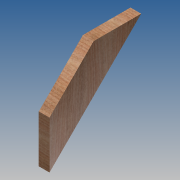
# Autodesk Inventor part: gableSupport
Saved by Autodesk Inventor 2013 (Build 170138000, 138)
## iProperties
Created: 2013-08-11
Part Number: gableSupport
Material: Wood (Birch)
Document SubType Name: Modeling
Designer: ddeboer
Mass: 2602.47 g
Surface Area: 2982.08 cm^2
Volume: 4731.76 cm^3
Density: 0.55 g/cm^3
Author: ddeboer
Autodesk Inventor part; units mm, degrees
ref_plane "YZ Plane" through (0, 0, 0) normal (1, 0, 0) x (0, 1, 0)
ref_plane "XZ Plane" through (0, 0, 0) normal (0, 1, 0) x (-1, 0, 0)
ref_plane "XY Plane" through (0, 0, 0) normal (0, 0, 1) x (1, 0, 0)
sketch "Sketch1" plane through (0, 0, 0) normal (1, 0, 0) x (0, 1, 0)
  line L0 (0, 0) -> (215.5261, -215.5261)
  line L1 (0, 0) -> (304.8, 0) construction
  line L2 (381, -183.4344) -> (337.2656, -139.7)
  line L3 (337.2656, -139.7) -> (197.5656, 0)
  line L4 (197.5656, 0) -> (0, 0)
  line L5 (215.5261, -215.5261) -> (381, -381)
  line L6 (381, -183.4344) -> (381, -381)
  dimension "d0" = 304.8
  dimension "d1" = 45
  dimension "d2" = 139.7
  dimension "d5" = 381
  constraints: 14 end point, 2 collinear, 1 equal length, 1 horizontal, 1 parallel, 1 perpendicular, 1 point on line
  measures "d0" distance of L0.start L0.end
  measures "d1" angle of L0 L1
  measures "d2" distance between parallel lines of L0 L2
  measures "d5" distance from line of L6 L0.start
extrude "Extrusion1" add sketch "Sketch1" along normal blind 44.45
body "Solid1"
